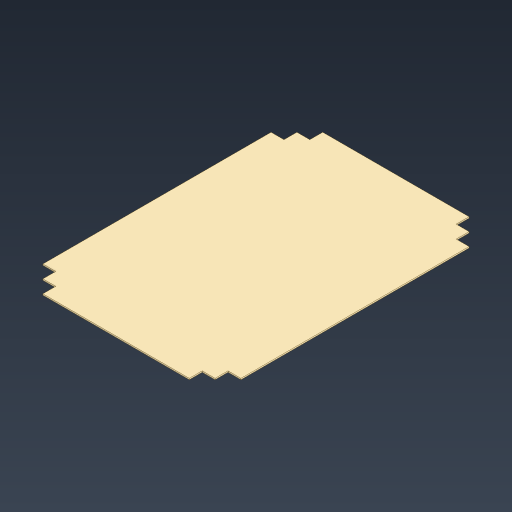
# Autodesk Inventor part: Фанера платформы
Saved by Autodesk Inventor 2023.2 (Build 272271030, 271C)
## iProperties
Created: 2025-08-21
Part Number: Фанера платформы
Material: Типовые
Document SubType Name: Modeling
Designer: Олег Коноваленко
Density: 1 g/cm^3
Appearance: Бежевый
Author: Олег Коноваленко
Autodesk Inventor part; units mm, degrees
ref_plane "YZ Plane" through (0, 0, 0) normal (1, 0, 0) x (0, 1, 0)
ref_plane "XZ Plane" through (0, 0, 0) normal (0, 1, 0) x (-1, 0, 0)
ref_plane "XY Plane" through (0, 0, 0) normal (0, 0, 1) x (1, 0, 0)
sketch "Эскиз1" plane through (0, 0, 0) normal (0, 1, 0) x (-1, 0, 0)
  line L0 (230, -325) -> (-230, -325)
  line L1 (-230, -325) -> (-230, 325)
  line L2 (-230, 325) -> (230, 325)
  line L3 (230, 325) -> (230, -325)
  line L4 (230, -325) -> (-230, 325) construction
  line L5 (-230, -325) -> (230, 325) construction
  line L6 (-230, -325) -> (-170, -325)
  line L7 (-170, -325) -> (-170, -295)
  line L8 (-170, -295) -> (-230, -295)
  line L9 (-230, -295) -> (-230, -325)
  line L10 (-230, -325) -> (-200, -325)
  line L11 (-200, -325) -> (-200, -265)
  line L12 (-200, -265) -> (-230, -265)
  line L13 (-230, -265) -> (-230, -325)
  line L14 (-230, 0) -> (230, 0) construction
  line L15 (0, -325) -> (0, 325) construction
  line L16 (-230, 325) -> (-170, 325)
  line L17 (-170, 325) -> (-170, 295)
  line L18 (-170, 295) -> (-230, 295)
  line L19 (-230, 295) -> (-230, 325)
  line L20 (-230, 325) -> (-200, 325)
  line L21 (-200, 325) -> (-200, 265)
  line L22 (-200, 265) -> (-230, 265)
  line L23 (-230, 265) -> (-230, 325)
  line L24 (230, -325) -> (170, -325)
  line L25 (170, -325) -> (170, -295)
  line L26 (170, -295) -> (230, -295)
  line L27 (230, -295) -> (230, -325)
  line L28 (230, -325) -> (200, -325)
  line L29 (200, -325) -> (200, -265)
  line L30 (200, -265) -> (230, -265)
  line L31 (230, -265) -> (230, -325)
  line L32 (170, 295) -> (230, 295)
  line L33 (230, 325) -> (170, 325)
  line L34 (170, 325) -> (170, 295)
  line L35 (230, 295) -> (230, 325)
  line L36 (230, 325) -> (200, 325)
  line L37 (200, 325) -> (200, 265)
  line L38 (230, 265) -> (230, 325)
  line L39 (200, 265) -> (230, 265)
  point P0 (0, 0)
  point P1 (200, 295)
  point P2 (-200, 295)
  point P3 (-200, -295)
  point P4 (200, -295)
  dimension "d0" = 650
  dimension "d1" = 460
  dimension "d2" = 30
  dimension "d3" = 60
  constraints: 80 end point, 18 symmetric about line, 6 midpoint, 6 parallel, 5 perpendicular, 3 horizontal
  measures "d0" distance of L0.end L1.end
  measures "d1" distance of L0.start L0.end
  measures "d2" distance of L6.end L7.end
  measures "d3" distance of L7.end L8.end
extrude "Выдавливание1" add sketch "Эскиз1" along normal blind 3 contours L0 L7 L8 L11 L12 L1 L22 L21 L18 L17 L2 L34 L32 L37 L39 L3 L30 L29 L26 L25
